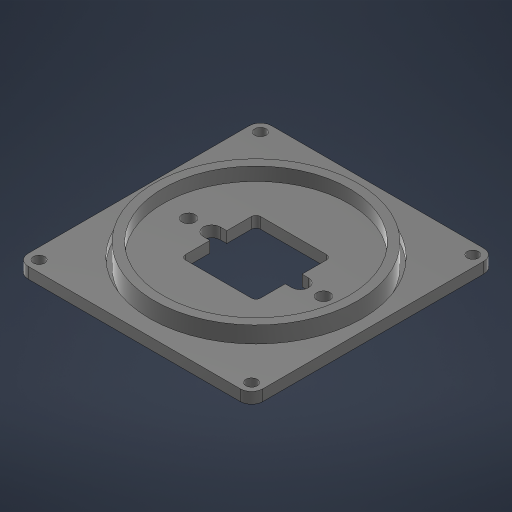
# Autodesk Inventor part: Camera_Mount
Saved by Autodesk Inventor 2024.2 (Build 282272000, 272)
## iProperties
Created: 2024-01-10
Part Number: Camera_Mount
Material: 一般
Document SubType Name: Modeling
Designer: Hanaoka
Density: 1 g/cm^3
Appearance: 既定
Author: Hanaoka
Autodesk Inventor part; units mm, degrees
ref_plane "YZ Plane" through (0, 0, 0) normal (1, 0, 0) x (0, 1, 0)
ref_plane "XZ Plane" through (0, 0, 0) normal (0, 1, 0) x (-1, 0, 0)
ref_plane "XY Plane" through (0, 0, 0) normal (0, 0, 1) x (1, 0, 0)
ref_plane "作業平面1" through (-1.8524, -8.2893, -39.454) normal (0, 1, 0) x (1, 0, 0)
sketch "スケッチ1" plane through (-1.8524, -8.2893, -39.454) normal (0, 1, 0) x (1, 0, 0)
  line L0 (9.655, 16.755) -> (9.655, 15.8775) projected
  arc A0 (6.855, 15.8775) -> (9.655, 15.8775) centre (8.255, 8.255) ccw projected
  line L1 (6.855, 15.8775) -> (6.855, 16.755) projected
  line L2 (6.855, 16.755) -> (0.755, 16.755) projected
  arc A1 (0.755, 16.755) -> (-0.245, 15.755) centre (0.755, 15.755) ccw projected
  line L3 (-0.245, 15.755) -> (-0.245, 10.155) projected
  line L4 (-0.245, 10.155) -> (-1.745, 10.155) projected
  arc A2 (-1.745, 10.155) -> (-1.745, 6.355) centre (-1.745, 8.255) ccw projected
  line L5 (-1.745, 6.355) -> (-0.245, 6.355) projected
  line L6 (-0.245, 6.355) -> (-0.245, 0.755) projected
  arc A3 (-0.245, 0.755) -> (0.755, -0.245) centre (0.755, 0.755) ccw projected
  line L7 (0.755, -0.245) -> (15.755, -0.245) projected
  arc A4 (15.755, -0.245) -> (16.755, 0.755) centre (15.755, 0.755) ccw projected
  line L8 (16.755, 0.755) -> (16.755, 6.355) projected
  line L9 (16.755, 6.355) -> (18.255, 6.355) projected
  arc A5 (18.255, 6.355) -> (18.255, 10.155) centre (18.255, 8.255) ccw projected
  line L10 (18.255, 10.155) -> (16.755, 10.155) projected
  line L11 (16.755, 10.155) -> (16.755, 15.755) projected
  arc A6 (16.755, 15.755) -> (15.755, 16.755) centre (15.755, 15.755) ccw projected
  line L12 (15.755, 16.755) -> (9.655, 16.755) projected
  circle A7 centre (-1.745, 8.255) radius 0.9 projected
  circle A8 centre (18.255, 8.255) radius 0.9 projected
  line L13 (-15.745, -19.245) -> (32.255, -19.245)
  line L14 (34.755, -16.745) -> (34.755, 33.255)
  line L15 (32.255, 35.755) -> (-15.745, 35.755)
  line L16 (-18.245, 33.255) -> (-18.245, -16.745)
  line L17 (-18.245, -19.245) -> (34.755, 35.755) construction
  line L18 (34.755, -19.245) -> (-18.245, 35.755) construction
  arc A9 (-15.745, 35.755) -> (-18.245, 33.255) centre (-15.745, 33.255) ccw
  arc A10 (34.755, 33.255) -> (32.255, 35.755) centre (32.255, 33.255) ccw
  arc A11 (32.255, -19.245) -> (34.755, -16.745) centre (32.255, -16.745) ccw
  arc A12 (-18.245, -16.745) -> (-15.745, -19.245) centre (-15.745, -16.745) ccw
  circle A13 centre (-15.745, 33.255) radius 1.3
  circle A14 centre (32.255, 33.255) radius 1.3
  circle A15 centre (32.255, -16.745) radius 1.3
  circle A16 centre (-15.745, -16.745) radius 1.3
  line L19 (32.255, -16.745) -> (-15.745, -16.745) construction
  line L20 (-15.745, -16.745) -> (-15.745, 33.255) construction
  line L21 (-15.745, 33.255) -> (32.255, 33.255) construction
  line L22 (32.255, 33.255) -> (32.255, -16.745) construction
  line L23 (32.255, -16.745) -> (-15.745, 33.255) construction
  line L24 (-15.745, -16.745) -> (32.255, 33.255) construction
  line L25 (6.855, 16.755) -> (9.655, 16.755)
  circle A17 centre (-6.985, 8.255) radius 1.5 projected
  circle A18 centre (18.26, 8.26) radius 1.27 projected
  circle A19 centre (23.495, 8.255) radius 1.5 projected
  point P0 (1.8524, -39.454)
  dimension "d2" = 2.5
  dimension "d3" = 2.6
  dimension "d4" = 50
  dimension "d5" = 48
  constraints: 26 end point, 8 centre point, 8 point on circle, 8 point on line, 8 tangent, 6 equal radius, 4 coincident, 4 midpoint, 4 parallel, 3 horizontal, 2 perpendicular
  measures "d2" radius of A9
  measures "d3" diameter of A14
  measures "d4" distance of L19.end L20.end
  measures "d5" distance of L20.end L21.end
extrude "押し出し1" add sketch "スケッチ1" along normal blind 2.5 contours A12 L16 A9 L15 A10 L14 A11 L13
sketch "スケッチ2" plane through (-1.8524, -5.7893, -39.454) normal (0, 1, 0) x (1, 0, 0)
  arc A0 (32.255, -19.245) -> (34.755, -16.745) centre (32.255, -16.745) ccw projected
  line L0 (34.755, -16.745) -> (34.755, 33.255) projected
  arc A1 (34.755, 33.255) -> (32.255, 35.755) centre (32.255, 33.255) ccw projected
  line L1 (32.255, 35.755) -> (-15.745, 35.755) projected
  arc A2 (-15.745, 35.755) -> (-18.245, 33.255) centre (-15.745, 33.255) ccw projected
  line L2 (-18.245, 33.255) -> (-18.245, -16.745) projected
  arc A3 (-18.245, -16.745) -> (-15.745, -19.245) centre (-15.745, -16.745) ccw projected
  line L3 (-15.745, -19.245) -> (32.255, -19.245) projected
  circle A4 centre (-15.745, -16.745) radius 1.3 projected
  circle A5 centre (32.255, -16.745) radius 1.3 projected
  circle A6 centre (32.255, 33.255) radius 1.3 projected
  circle A7 centre (-15.745, 33.255) radius 1.3 projected
  arc A8 (16.755, 15.755) -> (15.755, 16.755) centre (15.755, 15.755) ccw projected
  line L4 (16.755, 15.755) -> (16.755, 10.155) projected
  line L5 (16.755, 10.155) -> (18.255, 10.155) projected
  arc A9 (18.255, 6.355) -> (18.255, 10.155) centre (18.255, 8.255) ccw projected
  line L6 (18.255, 6.355) -> (16.755, 6.355) projected
  line L7 (16.755, 6.355) -> (16.755, 0.755) projected
  arc A10 (15.755, -0.245) -> (16.755, 0.755) centre (15.755, 0.755) ccw projected
  line L8 (15.755, -0.245) -> (0.755, -0.245) projected
  arc A11 (-0.245, 0.755) -> (0.755, -0.245) centre (0.755, 0.755) ccw projected
  line L9 (-0.245, 0.755) -> (-0.245, 6.355) projected
  line L10 (-0.245, 6.355) -> (-1.745, 6.355) projected
  arc A12 (-1.745, 10.155) -> (-1.745, 6.355) centre (-1.745, 8.255) ccw projected
  line L11 (-1.745, 10.155) -> (-0.245, 10.155) projected
  line L12 (-0.245, 10.155) -> (-0.245, 15.755) projected
  arc A13 (0.755, 16.755) -> (-0.245, 15.755) centre (0.755, 15.755) ccw projected
  line L13 (0.755, 16.755) -> (15.755, 16.755) projected
  circle A14 centre (8.255, 8.255) radius 24
  circle A15 centre (8.255, 8.255) radius 23
  circle A16 centre (8.255, 8.255) radius 21
  point P0 (1.8524, -39.454)
  dimension "d8" = 48
  dimension "d9" = 46
  dimension "d10" = 2
  constraints: 3 centre point, 2 coincident
  measures "d8" diameter of A14
  measures "d9" diameter of A15
  measures "d10" radial gap between concentric circles of A15 A16
extrude "押し出し2" add sketch "スケッチ2" along normal blind 3 contours A15
extrude "押し出し3" cut sketch "スケッチ2" against normal blind 2 contours A14
